Autodesk Fusion 360 part; units mm, degrees
(part 3 of 9)
sketch "Sketch4" plane through (0, 0, 11.2097) normal (0, 0, 1) x (-1, 0, 0)
  arc A0 (8.8437, -27.1341) -> (8.3894, -28.0773) centre (12.688, -29.5664) ccw
  arc A1 (7.8016, -28.4002) -> (8.3894, -28.0773) centre (7.917, -27.9137) ccw
  line L0 (7.8016, -28.4002) -> (6.2893, -28.0415)
  spline S0 degree 5 poles (6.2893, -28.0415) (6.2822, -28.0399) (6.268, -28.0368) (6.2464, -28.033) (6.2175, -28.0296) (6.181, -28.0275) (6.1441, -28.0271) (6.1072, -28.0276) (6.0701, -28.0286) (6.0329, -28.03) (5.9957, -28.0319) (5.9584, -28.0343) (5.921, -28.0374) (5.8835, -28.0413) (5.8459, -28.0461) (5.8083, -28.0516) (5.7706, -28.0577) (5.7328, -28.0644) (5.695, -28.0716) (5.6572, -28.0792) (5.6194, -28.0873) (5.5815, -28.0959) (5.5436, -28.1051) (5.5057, -28.1148) (5.4678, -28.125) (5.4299, -28.1357) (5.392, -28.1469) (5.354, -28.1586) (5.3161, -28.1707) (5.2782, -28.1833) (5.2403, -28.1963) (5.2024, -28.2097) (5.1646, -28.2236) (5.1267, -28.238) (5.0889, -28.2528) (5.0511, -28.268) (5.0134, -28.2837) (4.9757, -28.2998) (4.938, -28.3163) (4.9004, -28.3332) (4.8628, -28.3505) (4.8253, -28.3682) (4.7878, -28.3863) (4.7503, -28.4048) (4.713, -28.4238) (4.6756, -28.4431) (4.6384, -28.4628) (4.6012, -28.4829) (4.5641, -28.5034) (4.527, -28.5243) (4.49, -28.5455) (4.4531, -28.5672) (4.4163, -28.5892) (4.3795, -28.6115) (4.3429, -28.6343) (4.3063, -28.6574) (4.2698, -28.6809) (4.2334, -28.7048) (4.1971, -28.729) (4.1609, -28.7535) (4.1248, -28.7785) (4.0888, -28.8038) (4.0528, -28.8294) (4.017, -28.8554) (3.9813, -28.8817) (3.9457, -28.9084) (3.9102, -28.9354) (3.8749, -28.9628) (3.8396, -28.9905) (3.8045, -29.0186) (3.7695, -29.047) (3.7416, -29.0699) (3.7207, -29.0873) (3.7068, -29.099) (3.6998, -29.1048) knots 0 0 0 0 0 0 0.01428571 0.02857143 0.04285714 0.05714286 0.07142857 0.08571429 0.1 0.11428571 0.12857143 0.14285714 0.15714286 0.17142857 0.18571429 0.2 0.21428571 0.22857143 0.24285714 0.25714286 0.27142857 0.28571429 0.3 0.31428571 0.32857143 0.34285714 0.35714286 0.37142857 0.38571429 0.4 0.41428571 0.42857143 0.44285714 0.45714286 0.47142857 0.48571429 0.5 0.51428571 0.52857143 0.54285714 0.55714286 0.57142857 0.58571429 0.6 0.61428571 0.62857143 0.64285714 0.65714286 0.67142857 0.68571429 0.7 0.71428571 0.72857143 0.74285714 0.75714286 0.77142857 0.78571429 0.8 0.81428571 0.82857143 0.84285714 0.85714286 0.87142857 0.88571429 0.9 0.91428571 0.92857143 0.94285714 0.95714286 0.97142857 0.98571429 1 1 1 1 1 1
  arc A2 (3.6998, -29.1048) -> (3.6998, -30.028) centre (12.688, -29.5664) ccw
  spline S1 degree 5 poles (3.6998, -30.028) (3.7068, -30.0338) (3.7207, -30.0455) (3.7416, -30.0629) (3.7695, -30.0859) (3.8045, -30.1142) (3.8396, -30.1423) (3.8749, -30.17) (3.9102, -30.1974) (3.9457, -30.2244) (3.9813, -30.2511) (4.017, -30.2774) (4.0528, -30.3034) (4.0888, -30.3291) (4.1248, -30.3544) (4.1609, -30.3793) (4.1971, -30.4039) (4.2334, -30.4281) (4.2698, -30.4519) (4.3063, -30.4754) (4.3429, -30.4985) (4.3795, -30.5213) (4.4163, -30.5437) (4.4531, -30.5657) (4.49, -30.5873) (4.527, -30.6085) (4.5641, -30.6294) (4.6012, -30.6499) (4.6384, -30.67) (4.6756, -30.6897) (4.713, -30.709) (4.7503, -30.728) (4.7878, -30.7465) (4.8253, -30.7646) (4.8628, -30.7823) (4.9004, -30.7997) (4.938, -30.8166) (4.9757, -30.8331) (5.0134, -30.8491) (5.0511, -30.8648) (5.0889, -30.88) (5.1267, -30.8948) (5.1646, -30.9092) (5.2024, -30.9231) (5.2403, -30.9365) (5.2782, -30.9496) (5.3161, -30.9621) (5.354, -30.9742) (5.392, -30.9859) (5.4299, -30.9971) (5.4678, -31.0078) (5.5057, -31.0181) (5.5436, -31.0277) (5.5815, -31.0369) (5.6194, -31.0455) (5.6572, -31.0536) (5.695, -31.0613) (5.7328, -31.0684) (5.7706, -31.0751) (5.8083, -31.0812) (5.8459, -31.0867) (5.8835, -31.0915) (5.921, -31.0954) (5.9584, -31.0986) (5.9957, -31.101) (6.0329, -31.1028) (6.0701, -31.1042) (6.1072, -31.1053) (6.1441, -31.1058) (6.181, -31.1053) (6.2175, -31.1032) (6.2464, -31.0998) (6.268, -31.096) (6.2822, -31.093) (6.2893, -31.0913) knots -1 -1 -1 -1 -1 -1 -0.98571429 -0.97142857 -0.95714286 -0.94285714 -0.92857143 -0.91428571 -0.9 -0.88571429 -0.87142857 -0.85714286 -0.84285714 -0.82857143 -0.81428571 -0.8 -0.78571429 -0.77142857 -0.75714286 -0.74285714 -0.72857143 -0.71428571 -0.7 -0.68571429 -0.67142857 -0.65714286 -0.64285714 -0.62857143 -0.61428571 -0.6 -0.58571429 -0.57142857 -0.55714286 -0.54285714 -0.52857143 -0.51428571 -0.5 -0.48571429 -0.47142857 -0.45714286 -0.44285714 -0.42857143 -0.41428571 -0.4 -0.38571429 -0.37142857 -0.35714286 -0.34285714 -0.32857143 -0.31428571 -0.3 -0.28571429 -0.27142857 -0.25714286 -0.24285714 -0.22857143 -0.21428571 -0.2 -0.18571429 -0.17142857 -0.15714286 -0.14285714 -0.12857143 -0.11428571 -0.1 -0.08571429 -0.07142857 -0.05714286 -0.04285714 -0.02857143 -0.01428571 0 0 0 0 0 0
  line L1 (6.2893, -31.0913) -> (7.8016, -30.7327)
  arc A3 (8.3894, -31.0555) -> (7.8016, -30.7327) centre (7.917, -31.2192) ccw
  arc A4 (8.3894, -31.0555) -> (8.8437, -31.9987) centre (12.688, -29.5664) ccw
  arc A5 (8.7296, -32.6596) -> (8.8437, -31.9987) centre (8.4211, -32.2661) ccw
  line L2 (8.7296, -32.6596) -> (7.5063, -33.6183)
  spline S2 degree 5 poles (7.5063, -33.6183) (7.5006, -33.6229) (7.4893, -33.6321) (7.4729, -33.6466) (7.4522, -33.6671) (7.4278, -33.6943) (7.4045, -33.7228) (7.3818, -33.752) (7.3595, -33.7817) (7.3374, -33.8116) (7.3157, -33.8419) (7.2943, -33.8725) (7.2734, -33.9037) (7.2531, -33.9355) (7.2334, -33.9678) (7.2142, -34.0007) (7.1955, -34.034) (7.1772, -34.0677) (7.1592, -34.1017) (7.1416, -34.136) (7.1244, -34.1707) (7.1075, -34.2057) (7.091, -34.241) (7.075, -34.2767) (7.0593, -34.3127) (7.0441, -34.349) (7.0292, -34.3856) (7.0147, -34.4226) (7.0005, -34.4598) (6.9867, -34.4972) (6.9732, -34.535) (6.9601, -34.573) (6.9474, -34.6113) (6.935, -34.6498) (6.923, -34.6886) (6.9114, -34.7276) (6.9001, -34.7669) (6.8891, -34.8064) (6.8785, -34.8461) (6.8683, -34.8861) (6.8584, -34.9263) (6.8489, -34.9667) (6.8397, -35.0073) (6.8308, -35.0481) (6.8223, -35.0891) (6.8141, -35.1304) (6.8063, -35.1718) (6.7988, -35.2134) (6.7917, -35.2552) (6.7849, -35.2972) (6.7785, -35.3393) (6.7724, -35.3817) (6.7666, -35.4242) (6.7612, -35.4669) (6.7561, -35.5097) (6.7514, -35.5527) (6.747, -35.5959) (6.743, -35.6392) (6.7393, -35.6827) (6.7359, -35.7264) (6.7329, -35.7701) (6.7302, -35.8141) (6.7278, -35.8581) (6.7258, -35.9023) (6.7242, -35.9467) (6.7228, -35.9911) (6.7218, -36.0357) (6.7212, -36.0804) (6.7209, -36.1253) (6.7209, -36.1702) (6.7213, -36.2153) (6.7218, -36.2515) (6.7224, -36.2786) (6.7229, -36.2968) (6.7231, -36.3058) knots 0 0 0 0 0 0 0.01428571 0.02857143 0.04285714 0.05714286 0.07142857 0.08571429 0.1 0.11428571 0.12857143 0.14285714 0.15714286 0.17142857 0.18571429 0.2 0.21428571 0.22857143 0.24285714 0.25714286 0.27142857 0.28571429 0.3 0.31428571 0.32857143 0.34285714 0.35714286 0.37142857 0.38571429 0.4 0.41428571 0.42857143 0.44285714 0.45714286 0.47142857 0.48571429 0.5 0.51428571 0.52857143 0.54285714 0.55714286 0.57142857 0.58571429 0.6 0.61428571 0.62857143 0.64285714 0.65714286 0.67142857 0.68571429 0.7 0.71428571 0.72857143 0.74285714 0.75714286 0.77142857 0.78571429 0.8 0.81428571 0.82857143 0.84285714 0.85714286 0.87142857 0.88571429 0.9 0.91428571 0.92857143 0.94285714 0.95714286 0.97142857 0.98571429 1 1 1 1 1 1
  arc A6 (6.7231, -36.3058) -> (7.4448, -36.8814) centre (12.688, -29.5664) ccw
  spline S3 degree 5 poles (7.4448, -36.8814) (7.4537, -36.8796) (7.4715, -36.876) (7.4981, -36.8706) (7.5335, -36.8631) (7.5775, -36.8534) (7.6214, -36.8434) (7.665, -36.8331) (7.7085, -36.8225) (7.7517, -36.8117) (7.7948, -36.8005) (7.8376, -36.789) (7.8803, -36.7772) (7.9227, -36.7651) (7.9649, -36.7527) (8.007, -36.74) (8.0487, -36.727) (8.0903, -36.7137) (8.1317, -36.7001) (8.1728, -36.6862) (8.2137, -36.672) (8.2543, -36.6576) (8.2947, -36.6428) (8.3349, -36.6277) (8.3748, -36.6124) (8.4145, -36.5967) (8.4539, -36.5807) (8.4931, -36.5645) (8.532, -36.5479) (8.5706, -36.5311) (8.609, -36.514) (8.6471, -36.4966) (8.6849, -36.4788) (8.7225, -36.4608) (8.7597, -36.4425) (8.7967, -36.4239) (8.8334, -36.4051) (8.8698, -36.3859) (8.9058, -36.3664) (8.9416, -36.3467) (8.9771, -36.3266) (9.0122, -36.3063) (9.047, -36.2857) (9.0815, -36.2647) (9.1157, -36.2435) (9.1495, -36.222) (9.1829, -36.2002) (9.216, -36.1781) (9.2488, -36.1557) (9.2812, -36.1331) (9.3132, -36.1101) (9.3449, -36.0868) (9.3761, -36.0632) (9.4068, -36.0393) (9.4372, -36.0151) (9.4671, -35.9906) (9.4967, -35.9658) (9.5258, -35.9407) (9.5546, -35.9153) (9.5829, -35.8897) (9.6107, -35.8637) (9.6378, -35.8373) (9.6643, -35.8104) (9.69, -35.7831) (9.7152, -35.7554) (9.7398, -35.7275) (9.7641, -35.6993) (9.788, -35.671) (9.8115, -35.6424) (9.8341, -35.6133) (9.8552, -35.5835) (9.8706, -35.5587) (9.8811, -35.5395) (9.8876, -35.5264) (9.8907, -35.5198) knots -1 -1 -1 -1 -1 -1 -0.98571429 -0.97142857 -0.95714286 -0.94285714 -0.92857143 -0.91428571 -0.9 -0.88571429 -0.87142857 -0.85714286 -0.84285714 -0.82857143 -0.81428571 -0.8 -0.78571429 -0.77142857 -0.75714286 -0.74285714 -0.72857143 -0.71428571 -0.7 -0.68571429 -0.67142857 -0.65714286 -0.64285714 -0.62857143 -0.61428571 -0.6 -0.58571429 -0.57142857 -0.55714286 -0.54285714 -0.52857143 -0.51428571 -0.5 -0.48571429 -0.47142857 -0.45714286 -0.44285714 -0.42857143 -0.41428571 -0.4 -0.38571429 -0.37142857 -0.35714286 -0.34285714 -0.32857143 -0.31428571 -0.3 -0.28571429 -0.27142857 -0.25714286 -0.24285714 -0.22857143 -0.21428571 -0.2 -0.18571429 -0.17142857 -0.15714286 -0.14285714 -0.12857143 -0.11428571 -0.1 -0.08571429 -0.07142857 -0.05714286 -0.04285714 -0.02857143 -0.01428571 0 0 0 0 0 0
  line L3 (9.8907, -35.5198) -> (10.5532, -34.1139)
  arc A7 (11.1721, -33.8556) -> (10.5532, -34.1139) centre (11.0055, -34.327) ccw
  arc A8 (11.1721, -33.8556) -> (12.1928, -34.0886) centre (12.688, -29.5664) ccw
  arc A9 (12.6383, -34.5898) -> (12.1928, -34.0886) centre (12.1383, -34.5856) ccw
  line L4 (12.6383, -34.5898) -> (12.6252, -36.144)
  spline S4 degree 5 poles (12.6252, -36.144) (12.6251, -36.1513) (12.6253, -36.1659) (12.6264, -36.1877) (12.6295, -36.2167) (12.6357, -36.2527) (12.6434, -36.2887) (12.6521, -36.3247) (12.6614, -36.3606) (12.671, -36.3965) (12.6811, -36.4324) (12.6917, -36.4682) (12.7031, -36.504) (12.7153, -36.5397) (12.7283, -36.5752) (12.742, -36.6107) (12.7564, -36.6461) (12.7713, -36.6814) (12.7867, -36.7167) (12.8026, -36.7519) (12.8189, -36.7869) (12.8357, -36.8219) (12.8531, -36.8568) (12.871, -36.8916) (12.8893, -36.9263) (12.9082, -36.9609) (12.9276, -36.9954) (12.9474, -37.0298) (12.9677, -37.064) (12.9884, -37.0982) (13.0095, -37.1322) (13.031, -37.1662) (13.053, -37.2) (13.0754, -37.2337) (13.0983, -37.2673) (13.1215, -37.3007) (13.1452, -37.334) (13.1693, -37.3672) (13.1937, -37.4003) (13.2186, -37.4332) (13.2438, -37.466) (13.2694, -37.4986) (13.2955, -37.5312) (13.3219, -37.5635) (13.3486, -37.5958) (13.3758, -37.6278) (13.4033, -37.6598) (13.4312, -37.6916) (13.4594, -37.7232) (13.488, -37.7547) (13.5169, -37.786) (13.5462, -37.8172) (13.5759, -37.8482) (13.6059, -37.879) (13.6362, -37.9097) (13.6669, -37.9402) (13.6979, -37.9706) (13.7293, -38.0008) (13.761, -38.0308) (13.793, -38.0606) (13.8253, -38.0903) (13.858, -38.1198) (13.891, -38.1491) (13.9243, -38.1782) (13.9579, -38.2071) (13.9918, -38.2359) (14.0261, -38.2645) (14.0606, -38.2929) (14.0955, -38.3211) (14.1307, -38.3491) (14.1661, -38.3769) (14.1947, -38.399) (14.2163, -38.4155) (14.2308, -38.4265) (14.238, -38.4319) knots 0 0 0 0 0 0 0.01428571 0.02857143 0.04285714 0.05714286 0.07142857 0.08571429 0.1 0.11428571 0.12857143 0.14285714 0.15714286 0.17142857 0.18571429 0.2 0.21428571 0.22857143 0.24285714 0.25714286 0.27142857 0.28571429 0.3 0.31428571 0.32857143 0.34285714 0.35714286 0.37142857 0.38571429 0.4 0.41428571 0.42857143 0.44285714 0.45714286 0.47142857 0.48571429 0.5 0.51428571 0.52857143 0.54285714 0.55714286 0.57142857 0.58571429 0.6 0.61428571 0.62857143 0.64285714 0.65714286 0.67142857 0.68571429 0.7 0.71428571 0.72857143 0.74285714 0.75714286 0.77142857 0.78571429 0.8 0.81428571 0.82857143 0.84285714 0.85714286 0.87142857 0.88571429 0.9 0.91428571 0.92857143 0.94285714 0.95714286 0.97142857 0.98571429 1 1 1 1 1 1
  arc A10 (14.238, -38.4319) -> (15.1381, -38.2265) centre (12.688, -29.5664) ccw
  spline S5 degree 5 poles (15.1381, -38.2265) (15.1422, -38.2184) (15.1505, -38.2023) (15.1628, -38.1781) (15.179, -38.1457) (15.1989, -38.1053) (15.2184, -38.0648) (15.2376, -38.0243) (15.2564, -37.9837) (15.2748, -37.9431) (15.2929, -37.9024) (15.3107, -37.8618) (15.328, -37.8211) (15.345, -37.7803) (15.3617, -37.7396) (15.3779, -37.6988) (15.3938, -37.6581) (15.4094, -37.6173) (15.4245, -37.5765) (15.4393, -37.5357) (15.4537, -37.4949) (15.4677, -37.4541) (15.4814, -37.4133) (15.4946, -37.3725) (15.5075, -37.3317) (15.52, -37.2909) (15.5321, -37.2501) (15.5438, -37.2094) (15.5551, -37.1686) (15.5661, -37.1279) (15.5766, -37.0872) (15.5867, -37.0466) (15.5965, -37.006) (15.6058, -36.9654) (15.6147, -36.9249) (15.6232, -36.8844) (15.6313, -36.8439) (15.639, -36.8035) (15.6463, -36.7632) (15.6532, -36.7229) (15.6596, -36.6826) (15.6656, -36.6425) (15.6712, -36.6024) (15.6763, -36.5624) (15.681, -36.5225) (15.6853, -36.4826) (15.6891, -36.4429) (15.6925, -36.4032) (15.6954, -36.3637) (15.6979, -36.3242) (15.6999, -36.2848) (15.7015, -36.2456) (15.7025, -36.2065) (15.7029, -36.1675) (15.7029, -36.1287) (15.7024, -36.09) (15.7014, -36.0514) (15.7, -36.013) (15.6981, -35.9747) (15.6957, -35.9366) (15.6927, -35.8986) (15.689, -35.8609) (15.6845, -35.8235) (15.6792, -35.7864) (15.6732, -35.7494) (15.6668, -35.7127) (15.6599, -35.6762) (15.6526, -35.6398) (15.6449, -35.6037) (15.6362, -35.5679) (15.6261, -35.5327) (15.6163, -35.5052) (15.6079, -35.4851) (15.6017, -35.4719) (15.5985, -35.4653) knots -1 -1 -1 -1 -1 -1 -0.98571429 -0.97142857 -0.95714286 -0.94285714 -0.92857143 -0.91428571 -0.9 -0.88571429 -0.87142857 -0.85714286 -0.84285714 -0.82857143 -0.81428571 -0.8 -0.78571429 -0.77142857 -0.75714286 -0.74285714 -0.72857143 -0.71428571 -0.7 -0.68571429 -0.67142857 -0.65714286 -0.64285714 -0.62857143 -0.61428571 -0.6 -0.58571429 -0.57142857 -0.55714286 -0.54285714 -0.52857143 -0.51428571 -0.5 -0.48571429 -0.47142857 -0.45714286 -0.44285714 -0.42857143 -0.41428571 -0.4 -0.38571429 -0.37142857 -0.35714286 -0.34285714 -0.32857143 -0.31428571 -0.3 -0.28571429 -0.27142857 -0.25714286 -0.24285714 -0.22857143 -0.21428571 -0.2 -0.18571429 -0.17142857 -0.15714286 -0.14285714 -0.12857143 -0.11428571 -0.1 -0.08571429 -0.07142857 -0.05714286 -0.04285714 -0.02857143 -0.01428571 0 0 0 0 0 0
  line L5 (15.5985, -35.4653) -> (14.9123, -34.0708)
  arc A11 (15.0963, -33.4259) -> (14.9123, -34.0708) centre (15.361, -33.8501) ccw
  arc A12 (15.0963, -33.4259) -> (15.9148, -32.7731) centre (12.688, -29.5664) ccw
  arc A13 (16.5845, -32.7373) -> (15.9148, -32.7731) centre (16.2695, -33.1256) ccw
  line L6 (16.5845, -32.7373) -> (17.7914, -33.7165)
  spline S6 degree 5 poles (17.7914, -33.7165) (17.7971, -33.7211) (17.8086, -33.7301) (17.8263, -33.7429) (17.8509, -33.7585) (17.8829, -33.7762) (17.9159, -33.7926) (17.9494, -33.8082) (17.9833, -33.8233) (18.0174, -33.8382) (18.0517, -33.8527) (18.0864, -33.8667) (18.1214, -33.8801) (18.1569, -33.8928) (18.1928, -33.9048) (18.2292, -33.9162) (18.2658, -33.9271) (18.3027, -33.9374) (18.3399, -33.9474) (18.3772, -33.9569) (18.4149, -33.966) (18.4527, -33.9746) (18.4908, -33.9828) (18.5292, -33.9906) (18.5677, -33.9978) (18.6066, -34.0046) (18.6456, -34.011) (18.6848, -34.0169) (18.7243, -34.0224) (18.7639, -34.0276) (18.8037, -34.0323) (18.8436, -34.0366) (18.8838, -34.0405) (18.9241, -34.044) (18.9646, -34.047) (19.0052, -34.0497) (19.046, -34.052) (19.087, -34.0539) (19.1281, -34.0554) (19.1693, -34.0565) (19.2107, -34.0572) (19.2522, -34.0575) (19.2938, -34.0574) (19.3356, -34.057) (19.3775, -34.0561) (19.4195, -34.0549) (19.4616, -34.0533) (19.5039, -34.0513) (19.5462, -34.049) (19.5886, -34.0463) (19.6312, -34.0432) (19.6738, -34.0397) (19.7165, -34.0358) (19.7594, -34.0316) (19.8023, -34.027) (19.8453, -34.0221) (19.8883, -34.0167) (19.9315, -34.011) (19.9747, -34.005) (20.018, -33.9986) (20.0613, -33.9918) (20.1047, -33.9846) (20.1482, -33.9771) (20.1918, -33.9692) (20.2354, -33.961) (20.279, -33.9524) (20.3227, -33.9434) (20.3664, -33.9341) (20.4102, -33.9244) (20.4541, -33.9144) (20.4979, -33.904) (20.533, -33.8954) (20.5594, -33.8888) (20.577, -33.8843) (20.5858, -33.8821) knots 0 0 0 0 0 0 0.01428571 0.02857143 0.04285714 0.05714286 0.07142857 0.08571429 0.1 0.11428571 0.12857143 0.14285714 0.15714286 0.17142857 0.18571429 0.2 0.21428571 0.22857143 0.24285714 0.25714286 0.27142857 0.28571429 0.3 0.31428571 0.32857143 0.34285714 0.35714286 0.37142857 0.38571429 0.4 0.41428571 0.42857143 0.44285714 0.45714286 0.47142857 0.48571429 0.5 0.51428571 0.52857143 0.54285714 0.55714286 0.57142857 0.58571429 0.6 0.61428571 0.62857143 0.64285714 0.65714286 0.67142857 0.68571429 0.7 0.71428571 0.72857143 0.74285714 0.75714286 0.77142857 0.78571429 0.8 0.81428571 0.82857143 0.84285714 0.85714286 0.87142857 0.88571429 0.9 0.91428571 0.92857143 0.94285714 0.95714286 0.97142857 0.98571429 1 1 1 1 1 1
  arc A14 (20.5858, -33.8821) -> (20.9863, -33.0504) centre (12.688, -29.5664) ccw
  spline S7 degree 5 poles (20.9863, -33.0504) (20.9826, -33.0421) (20.9751, -33.0255) (20.9639, -33.0008) (20.9487, -32.968) (20.9295, -32.9272) (20.91, -32.8867) (20.8902, -32.8465) (20.8702, -32.8064) (20.85, -32.7667) (20.8295, -32.7272) (20.8088, -32.688) (20.7878, -32.649) (20.7666, -32.6104) (20.7451, -32.5719) (20.7234, -32.5338) (20.7014, -32.496) (20.6792, -32.4584) (20.6567, -32.4211) (20.634, -32.3841) (20.6111, -32.3474) (20.588, -32.311) (20.5646, -32.2749) (20.5409, -32.2391) (20.5171, -32.2036) (20.493, -32.1684) (20.4686, -32.1335) (20.4441, -32.0989) (20.4193, -32.0647) (20.3943, -32.0308) (20.369, -31.9972) (20.3436, -31.9639) (20.3179, -31.931) (20.292, -31.8984) (20.2658, -31.8661) (20.2395, -31.8342) (20.2129, -31.8027) (20.1861, -31.7714) (20.1591, -31.7406) (20.1319, -31.7101) (20.1045, -31.68) (20.0768, -31.6503) (20.049, -31.6209) (20.0209, -31.592) (19.9926, -31.5634) (19.9641, -31.5352) (19.9354, -31.5075) (19.9065, -31.4801) (19.8774, -31.4531) (19.8481, -31.4266) (19.8186, -31.4004) (19.7888, -31.3748) (19.7589, -31.3496) (19.7287, -31.3249) (19.6984, -31.3008) (19.6678, -31.277) (19.637, -31.2537) (19.6061, -31.2309) (19.575, -31.2085) (19.5437, -31.1866) (19.5121, -31.1653) (19.4803, -31.1447) (19.4483, -31.1249) (19.4159, -31.1059) (19.3834, -31.0875) (19.3506, -31.0697) (19.3178, -31.0523) (19.2848, -31.0353) (19.2517, -31.0188) (19.2183, -31.0032) (19.1845, -30.9892) (19.157, -30.9797) (19.1359, -30.9738) (19.1217, -30.9704) (19.1146, -30.9688) knots -1 -1 -1 -1 -1 -1 -0.98571429 -0.97142857 -0.95714286 -0.94285714 -0.92857143 -0.91428571 -0.9 -0.88571429 -0.87142857 -0.85714286 -0.84285714 -0.82857143 -0.81428571 -0.8 -0.78571429 -0.77142857 -0.75714286 -0.74285714 -0.72857143 -0.71428571 -0.7 -0.68571429 -0.67142857 -0.65714286 -0.64285714 -0.62857143 -0.61428571 -0.6 -0.58571429 -0.57142857 -0.55714286 -0.54285714 -0.52857143 -0.51428571 -0.5 -0.48571429 -0.47142857 -0.45714286 -0.44285714 -0.42857143 -0.41428571 -0.4 -0.38571429 -0.37142857 -0.35714286 -0.34285714 -0.32857143 -0.31428571 -0.3 -0.28571429 -0.27142857 -0.25714286 -0.24285714 -0.22857143 -0.21428571 -0.2 -0.18571429 -0.17142857 -0.15714286 -0.14285714 -0.12857143 -0.11428571 -0.1 -0.08571429 -0.07142857 -0.05714286 -0.04285714 -0.02857143 -0.01428571 0 0 0 0 0 0
  line L7 (19.1146, -30.9688) -> (17.5965, -30.6358)
  arc A15 (17.207, -30.0899) -> (17.5965, -30.6358) centre (17.7037, -30.1474) ccw
  arc A16 (17.207, -30.0899) -> (17.207, -29.0429) centre (12.688, -29.5664) ccw
  arc A17 (17.5965, -28.497) -> (17.207, -29.0429) centre (17.7037, -28.9854) ccw
  line L8 (17.5965, -28.497) -> (19.1146, -28.164)
  spline S8 degree 5 poles (19.1146, -28.164) (19.1217, -28.1624) (19.1359, -28.159) (19.157, -28.1531) (19.1845, -28.1436) (19.2183, -28.1296) (19.2517, -28.114) (19.2848, -28.0976) (19.3178, -28.0805) (19.3506, -28.0631) (19.3834, -28.0453) (19.4159, -28.027) (19.4483, -28.0079) (19.4803, -27.9881) (19.5121, -27.9675) (19.5437, -27.9462) (19.575, -27.9243) (19.6061, -27.9019) (19.637, -27.8791) (19.6678, -27.8558) (19.6984, -27.8321) (19.7287, -27.8079) (19.7589, -27.7832) (19.7888, -27.758) (19.8186, -27.7324) (19.8481, -27.7063) (19.8774, -27.6797) (19.9065, -27.6527) (19.9354, -27.6254) (19.9641, -27.5976) (19.9926, -27.5694) (20.0209, -27.5409) (20.049, -27.5119) (20.0768, -27.4826) (20.1045, -27.4528) (20.1319, -27.4227) (20.1591, -27.3922) (20.1861, -27.3614) (20.2129, -27.3302) (20.2395, -27.2986) (20.2658, -27.2667) (20.292, -27.2344) (20.3179, -27.2019) (20.3436, -27.1689) (20.369, -27.1356) (20.3943, -27.102) (20.4193, -27.0681) (20.4441, -27.0339) (20.4686, -26.9993) (20.493, -26.9644) (20.5171, -26.9292) (20.5409, -26.8937) (20.5646, -26.8579) (20.588, -26.8218) (20.6111, -26.7854) (20.634, -26.7487) (20.6567, -26.7117) (20.6792, -26.6744) (20.7014, -26.6369) (20.7234, -26.599) (20.7451, -26.5609) (20.7666, -26.5225) (20.7878, -26.4838) (20.8088, -26.4448) (20.8295, -26.4056) (20.85, -26.3661) (20.8702, -26.3264) (20.8902, -26.2864) (20.91, -26.2461) (20.9295, -26.2056) (20.9487, -26.1648) (20.9639, -26.132) (20.9751, -26.1073) (20.9826, -26.0907) (20.9863, -26.0825) knots 0 0 0 0 0 0 0.01428571 0.02857143 0.04285714 0.05714286 0.07142857 0.08571429 0.1 0.11428571 0.12857143 0.14285714 0.15714286 0.17142857 0.18571429 0.2 0.21428571 0.22857143 0.24285714 0.25714286 0.27142857 0.28571429 0.3 0.31428571 0.32857143 0.34285714 0.35714286 0.37142857 0.38571429 0.4 0.41428571 0.42857143 0.44285714 0.45714286 0.47142857 0.48571429 0.5 0.51428571 0.52857143 0.54285714 0.55714286 0.57142857 0.58571429 0.6 0.61428571 0.62857143 0.64285714 0.65714286 0.67142857 0.68571429 0.7 0.71428571 0.72857143 0.74285714 0.75714286 0.77142857 0.78571429 0.8 0.81428571 0.82857143 0.84285714 0.85714286 0.87142857 0.88571429 0.9 0.91428571 0.92857143 0.94285714 0.95714286 0.97142857 0.98571429 1 1 1 1 1 1
  arc A18 (20.9863, -26.0825) -> (20.5858, -25.2507) centre (12.688, -29.5664) ccw
  spline S9 degree 5 poles (20.5858, -25.2507) (20.577, -25.2485) (20.5594, -25.244) (20.533, -25.2374) (20.4979, -25.2288) (20.4541, -25.2184) (20.4102, -25.2084) (20.3664, -25.1987) (20.3227, -25.1894) (20.279, -25.1804) (20.2354, -25.1718) (20.1918, -25.1636) (20.1482, -25.1557) (20.1047, -25.1482) (20.0613, -25.1411) (20.018, -25.1343) (19.9747, -25.1278) (19.9315, -25.1218) (19.8883, -25.1161) (19.8453, -25.1108) (19.8023, -25.1058) (19.7594, -25.1012) (19.7165, -25.097) (19.6738, -25.0931) (19.6312, -25.0897) (19.5886, -25.0866) (19.5462, -25.0838) (19.5039, -25.0815) (19.4616, -25.0795) (19.4195, -25.0779) (19.3775, -25.0767) (19.3356, -25.0759) (19.2938, -25.0754) (19.2522, -25.0753) (19.2107, -25.0757) (19.1693, -25.0764) (19.1281, -25.0775) (19.087, -25.079) (19.046, -25.0808) (19.0052, -25.0831) (18.9646, -25.0858) (18.9241, -25.0889) (18.8838, -25.0923) (18.8436, -25.0962) (18.8037, -25.1005) (18.7639, -25.1053) (18.7243, -25.1104) (18.6848, -25.1159) (18.6456, -25.1218) (18.6066, -25.1282) (18.5677, -25.135) (18.5292, -25.1423) (18.4908, -25.15) (18.4527, -25.1582) (18.4149, -25.1668) (18.3772, -25.1759) (18.3399, -25.1855) (18.3027, -25.1954) (18.2658, -25.2058) (18.2292, -25.2166) (18.1928, -25.228) (18.1569, -25.24) (18.1214, -25.2527) (18.0864, -25.2661) (18.0517, -25.2801) (18.0174, -25.2946) (17.9833, -25.3095) (17.9494, -25.3246) (17.9159, -25.3402) (17.8829, -25.3566) (17.8509, -25.3743) (17.8263, -25.39) (17.8086, -25.4027) (17.7971, -25.4117) (17.7914, -25.4163) knots -1 -1 -1 -1 -1 -1 -0.98571429 -0.97142857 -0.95714286 -0.94285714 -0.92857143 -0.91428571 -0.9 -0.88571429 -0.87142857 -0.85714286 -0.84285714 -0.82857143 -0.81428571 -0.8 -0.78571429 -0.77142857 -0.75714286 -0.74285714 -0.72857143 -0.71428571 -0.7 -0.68571429 -0.67142857 -0.65714286 -0.64285714 -0.62857143 -0.61428571 -0.6 -0.58571429 -0.57142857 -0.55714286 -0.54285714 -0.52857143 -0.51428571 -0.5 -0.48571429 -0.47142857 -0.45714286 -0.44285714 -0.42857143 -0.41428571 -0.4 -0.38571429 -0.37142857 -0.35714286 -0.34285714 -0.32857143 -0.31428571 -0.3 -0.28571429 -0.27142857 -0.25714286 -0.24285714 -0.22857143 -0.21428571 -0.2 -0.18571429 -0.17142857 -0.15714286 -0.14285714 -0.12857143 -0.11428571 -0.1 -0.08571429 -0.07142857 -0.05714286 -0.04285714 -0.02857143 -0.01428571 0 0 0 0 0 0
  line L9 (17.7914, -25.4163) -> (16.5845, -26.3955)
  arc A19 (15.9148, -26.3597) -> (16.5845, -26.3955) centre (16.2695, -26.0073) ccw
  arc A20 (15.9148, -26.3597) -> (15.0963, -25.707) centre (12.688, -29.5664) ccw
  arc A21 (14.9123, -25.062) -> (15.0963, -25.707) centre (15.361, -25.2828) ccw
  line L10 (14.9123, -25.062) -> (15.5985, -23.6675)
  spline S10 degree 5 poles (15.5985, -23.6675) (15.6017, -23.6609) (15.6079, -23.6477) (15.6163, -23.6276) (15.6261, -23.6001) (15.6362, -23.5649) (15.6449, -23.5292) (15.6526, -23.493) (15.6599, -23.4566) (15.6668, -23.4201) (15.6732, -23.3834) (15.6792, -23.3465) (15.6845, -23.3093) (15.689, -23.2719) (15.6927, -23.2342) (15.6957, -23.1963) (15.6981, -23.1581) (15.7, -23.1198) (15.7014, -23.0814) (15.7024, -23.0428) (15.7029, -23.0041) (15.7029, -22.9653) (15.7025, -22.9263) (15.7015, -22.8872) (15.6999, -22.848) (15.6979, -22.8086) (15.6954, -22.7692) (15.6925, -22.7296) (15.6891, -22.6899) (15.6853, -22.6502) (15.681, -22.6103) (15.6763, -22.5704) (15.6712, -22.5304) (15.6656, -22.4903) (15.6596, -22.4502) (15.6532, -22.4099) (15.6463, -22.3697) (15.639, -22.3293) (15.6313, -22.2889) (15.6232, -22.2485) (15.6147, -22.208) (15.6058, -22.1674) (15.5965, -22.1268) (15.5867, -22.0862) (15.5766, -22.0456) (15.5661, -22.0049) (15.5551, -21.9642) (15.5438, -21.9235) (15.5321, -21.8827) (15.52, -21.8419) (15.5075, -21.8011) (15.4946, -21.7604) (15.4814, -21.7195) (15.4677, -21.6787) (15.4537, -21.6379) (15.4393, -21.5971) (15.4245, -21.5563) (15.4094, -21.5155) (15.3938, -21.4747) (15.3779, -21.434) (15.3617, -21.3932) (15.345, -21.3525) (15.328, -21.3118) (15.3107, -21.2711) (15.2929, -21.2304) (15.2748, -21.1897) (15.2564, -21.1491) (15.2376, -21.1086) (15.2184, -21.068) (15.1989, -21.0275) (15.179, -20.9871) (15.1628, -20.9548) (15.1505, -20.9305) (15.1422, -20.9144) (15.1381, -20.9063) knots 0 0 0 0 0 0 0.01428571 0.02857143 0.04285714 0.05714286 0.07142857 0.08571429 0.1 0.11428571 0.12857143 0.14285714 0.15714286 0.17142857 0.18571429 0.2 0.21428571 0.22857143 0.24285714 0.25714286 0.27142857 0.28571429 0.3 0.31428571 0.32857143 0.34285714 0.35714286 0.37142857 0.38571429 0.4 0.41428571 0.42857143 0.44285714 0.45714286 0.47142857 0.48571429 0.5 0.51428571 0.52857143 0.54285714 0.55714286 0.57142857 0.58571429 0.6 0.61428571 0.62857143 0.64285714 0.65714286 0.67142857 0.68571429 0.7 0.71428571 0.72857143 0.74285714 0.75714286 0.77142857 0.78571429 0.8 0.81428571 0.82857143 0.84285714 0.85714286 0.87142857 0.88571429 0.9 0.91428571 0.92857143 0.94285714 0.95714286 0.97142857 0.98571429 1 1 1 1 1 1
  arc A22 (15.1381, -20.9063) -> (14.238, -20.7009) centre (12.688, -29.5664) ccw
  spline S11 degree 5 poles (14.238, -20.7009) (14.2308, -20.7064) (14.2163, -20.7173) (14.1947, -20.7338) (14.1661, -20.7559) (14.1307, -20.7837) (14.0955, -20.8117) (14.0606, -20.8399) (14.0261, -20.8683) (13.9918, -20.8969) (13.9579, -20.9257) (13.9243, -20.9546) (13.891, -20.9837) (13.858, -21.0131) (13.8253, -21.0425) (13.793, -21.0722) (13.761, -21.102) (13.7293, -21.1321) (13.6979, -21.1622) (13.6669, -21.1926) (13.6362, -21.2231) (13.6059, -21.2538) (13.5759, -21.2846) (13.5462, -21.3156) (13.5169, -21.3468) (13.488, -21.3781) (13.4594, -21.4096) (13.4312, -21.4412) (13.4033, -21.473) (13.3758, -21.505) (13.3486, -21.5371) (13.3219, -21.5693) (13.2955, -21.6017) (13.2694, -21.6342) (13.2438, -21.6668) (13.2186, -21.6996) (13.1937, -21.7325) (13.1693, -21.7656) (13.1452, -21.7988) (13.1215, -21.8321) (13.0983, -21.8656) (13.0754, -21.8991) (13.053, -21.9328) (13.031, -21.9666) (13.0095, -22.0006) (12.9884, -22.0346) (12.9677, -22.0688) (12.9474, -22.103) (12.9276, -22.1374) (12.9082, -22.1719) (12.8893, -22.2065) (12.871, -22.2412) (12.8531, -22.276) (12.8357, -22.3109) (12.8189, -22.3459) (12.8026, -22.381) (12.7867, -22.4161) (12.7713, -22.4514) (12.7564, -22.4867) (12.742, -22.5221) (12.7283, -22.5576) (12.7153, -22.5932) (12.7031, -22.6288) (12.6917, -22.6646) (12.6811, -22.7004) (12.671, -22.7363) (12.6614, -22.7722) (12.6521, -22.8082) (12.6434, -22.8441) (12.6357, -22.8801) (12.6295, -22.9162) (12.6264, -22.9451) (12.6253, -22.967) (12.6251, -22.9816) (12.6252, -22.9889) knots -1 -1 -1 -1 -1 -1 -0.98571429 -0.97142857 -0.95714286 -0.94285714 -0.92857143 -0.91428571 -0.9 -0.88571429 -0.87142857 -0.85714286 -0.84285714 -0.82857143 -0.81428571 -0.8 -0.78571429 -0.77142857 -0.75714286 -0.74285714 -0.72857143 -0.71428571 -0.7 -0.68571429 -0.67142857 -0.65714286 -0.64285714 -0.62857143 -0.61428571 -0.6 -0.58571429 -0.57142857 -0.55714286 -0.54285714 -0.52857143 -0.51428571 -0.5 -0.48571429 -0.47142857 -0.45714286 -0.44285714 -0.42857143 -0.41428571 -0.4 -0.38571429 -0.37142857 -0.35714286 -0.34285714 -0.32857143 -0.31428571 -0.3 -0.28571429 -0.27142857 -0.25714286 -0.24285714 -0.22857143 -0.21428571 -0.2 -0.18571429 -0.17142857 -0.15714286 -0.14285714 -0.12857143 -0.11428571 -0.1 -0.08571429 -0.07142857 -0.05714286 -0.04285714 -0.02857143 -0.01428571 0 0 0 0 0 0
  line L11 (12.6252, -22.9889) -> (12.6383, -24.543)
  arc A23 (12.1928, -25.0442) -> (12.6383, -24.543) centre (12.1383, -24.5472) ccw
  arc A24 (12.1928, -25.0442) -> (11.1721, -25.2772) centre (12.688, -29.5664) ccw
  arc A25 (10.5532, -25.0189) -> (11.1721, -25.2772) centre (11.0055, -24.8058) ccw
  line L12 (10.5532, -25.0189) -> (9.8907, -23.613)
  spline S12 degree 5 poles (9.8907, -23.613) (9.8876, -23.6064) (9.8811, -23.5933) (9.8706, -23.5741) (9.8552, -23.5494) (9.8341, -23.5195) (9.8115, -23.4905) (9.788, -23.4619) (9.7641, -23.4335) (9.7398, -23.4053) (9.7152, -23.3774) (9.69, -23.3497) (9.6643, -23.3224) (9.6378, -23.2956) (9.6107, -23.2692) (9.5829, -23.2431) (9.5546, -23.2175) (9.5258, -23.1921) (9.4967, -23.1671) (9.4671, -23.1423) (9.4372, -23.1177) (9.4068, -23.0935) (9.3761, -23.0696) (9.3449, -23.046) (9.3132, -23.0227) (9.2812, -22.9998) (9.2488, -22.9771) (9.216, -22.9547) (9.1829, -22.9326) (9.1495, -22.9108) (9.1157, -22.8893) (9.0815, -22.8681) (9.047, -22.8472) (9.0122, -22.8265) (8.9771, -22.8062) (8.9416, -22.7862) (8.9058, -22.7664) (8.8698, -22.7469) (8.8334, -22.7278) (8.7967, -22.7089) (8.7597, -22.6903) (8.7225, -22.672) (8.6849, -22.654) (8.6471, -22.6363) (8.609, -22.6188) (8.5706, -22.6017) (8.532, -22.5849) (8.4931, -22.5683) (8.4539, -22.5521) (8.4145, -22.5361) (8.3748, -22.5205) (8.3349, -22.5051) (8.2947, -22.49) (8.2543, -22.4752) (8.2137, -22.4608) (8.1728, -22.4466) (8.1317, -22.4327) (8.0903, -22.4191) (8.0487, -22.4058) (8.007, -22.3928) (7.9649, -22.3801) (7.9227, -22.3677) (7.8803, -22.3556) (7.8376, -22.3439) (7.7948, -22.3324) (7.7517, -22.3212) (7.7085, -22.3103) (7.665, -22.2997) (7.6214, -22.2894) (7.5775, -22.2794) (7.5335, -22.2698) (7.4981, -22.2623) (7.4715, -22.2568) (7.4537, -22.2532) (7.4448, -22.2514) knots 0 0 0 0 0 0 0.01428571 0.02857143 0.04285714 0.05714286 0.07142857 0.08571429 0.1 0.11428571 0.12857143 0.14285714 0.15714286 0.17142857 0.18571429 0.2 0.21428571 0.22857143 0.24285714 0.25714286 0.27142857 0.28571429 0.3 0.31428571 0.32857143 0.34285714 0.35714286 0.37142857 0.38571429 0.4 0.41428571 0.42857143 0.44285714 0.45714286 0.47142857 0.48571429 0.5 0.51428571 0.52857143 0.54285714 0.55714286 0.57142857 0.58571429 0.6 0.61428571 0.62857143 0.64285714 0.65714286 0.67142857 0.68571429 0.7 0.71428571 0.72857143 0.74285714 0.75714286 0.77142857 0.78571429 0.8 0.81428571 0.82857143 0.84285714 0.85714286 0.87142857 0.88571429 0.9 0.91428571 0.92857143 0.94285714 0.95714286 0.97142857 0.98571429 1 1 1 1 1 1
  arc A26 (7.4448, -22.2514) -> (6.7231, -22.827) centre (12.688, -29.5664) ccw
  spline S13 degree 5 poles (6.7231, -22.827) (6.7229, -22.836) (6.7224, -22.8542) (6.7218, -22.8813) (6.7213, -22.9175) (6.7209, -22.9626) (6.7209, -23.0075) (6.7212, -23.0524) (6.7218, -23.0971) (6.7228, -23.1417) (6.7242, -23.1862) (6.7258, -23.2305) (6.7278, -23.2747) (6.7302, -23.3188) (6.7329, -23.3627) (6.7359, -23.4065) (6.7393, -23.4501) (6.743, -23.4936) (6.747, -23.5369) (6.7514, -23.5801) (6.7561, -23.6231) (6.7612, -23.6659) (6.7666, -23.7086) (6.7724, -23.7511) (6.7785, -23.7935) (6.7849, -23.8357) (6.7917, -23.8776) (6.7988, -23.9194) (6.8063, -23.961) (6.8141, -24.0025) (6.8223, -24.0437) (6.8308, -24.0847) (6.8397, -24.1255) (6.8489, -24.1661) (6.8584, -24.2065) (6.8683, -24.2467) (6.8785, -24.2867) (6.8891, -24.3264) (6.9001, -24.3659) (6.9114, -24.4052) (6.923, -24.4442) (6.935, -24.483) (6.9474, -24.5216) (6.9601, -24.5598) (6.9732, -24.5978) (6.9867, -24.6356) (7.0005, -24.6731) (7.0147, -24.7103) (7.0292, -24.7472) (7.0441, -24.7838) (7.0593, -24.8202) (7.075, -24.8562) (7.091, -24.8918) (7.1075, -24.9272) (7.1244, -24.9621) (7.1416, -24.9968) (7.1592, -25.0311) (7.1772, -25.0651) (7.1955, -25.0988) (7.2142, -25.1321) (7.2334, -25.165) (7.2531, -25.1973) (7.2734, -25.2291) (7.2943, -25.2603) (7.3157, -25.2909) (7.3374, -25.3212) (7.3595, -25.3511) (7.3818, -25.3808) (7.4045, -25.41) (7.4278, -25.4385) (7.4522, -25.4658) (7.4729, -25.4863) (7.4893, -25.5007) (7.5006, -25.51) (7.5063, -25.5145) knots -1 -1 -1 -1 -1 -1 -0.98571429 -0.97142857 -0.95714286 -0.94285714 -0.92857143 -0.91428571 -0.9 -0.88571429 -0.87142857 -0.85714286 -0.84285714 -0.82857143 -0.81428571 -0.8 -0.78571429 -0.77142857 -0.75714286 -0.74285714 -0.72857143 -0.71428571 -0.7 -0.68571429 -0.67142857 -0.65714286 -0.64285714 -0.62857143 -0.61428571 -0.6 -0.58571429 -0.57142857 -0.55714286 -0.54285714 -0.52857143 -0.51428571 -0.5 -0.48571429 -0.47142857 -0.45714286 -0.44285714 -0.42857143 -0.41428571 -0.4 -0.38571429 -0.37142857 -0.35714286 -0.34285714 -0.32857143 -0.31428571 -0.3 -0.28571429 -0.27142857 -0.25714286 -0.24285714 -0.22857143 -0.21428571 -0.2 -0.18571429 -0.17142857 -0.15714286 -0.14285714 -0.12857143 -0.11428571 -0.1 -0.08571429 -0.07142857 -0.05714286 -0.04285714 -0.02857143 -0.01428571 0 0 0 0 0 0
  line L13 (7.5063, -25.5145) -> (8.7296, -26.4732)
  arc A27 (8.8437, -27.1341) -> (8.7296, -26.4732) centre (8.4211, -26.8667) ccw
  circle A28 centre (12.688, -29.5664) radius 2.5
  line L14 (15.1873, -29.6249) -> (10.188, -29.5664)
  line L15 (15.1873, -29.6249) -> (10.6876, -29.5723)
  line L16 (10.6876, -29.5723) -> (10.7055, -28.0434)
  line L17 (10.7055, -28.0434) -> (10.6876, -29.5723)
  line L18 (10.6876, -29.5723) -> (10.6704, -31.0427)
  dimension "d66" = 4.5
  constraint coincident A28 L14.start
  constraint coincident A28 L14.end
  constraint parallel L14 L15
  constraint coincident A28 L16.end
  constraint perpendicular L15 L16
  constraint coincident A28 L18.end
  constraint perpendicular L14 L18
  measures "d66" distance of L14.start L15.end
extrude "Extrude5" add sketch "Sketch4" against normal blind 11.5 contours A28 L14 L16 L17 | A28 L14 L18 sketch seen with x (1, 0, 0) y (0, 1, 0) z (0, 0, 1) at (12.688, -29.5664, 0.2903) bodies 5 in component "Spur Gear (7 teeth)"